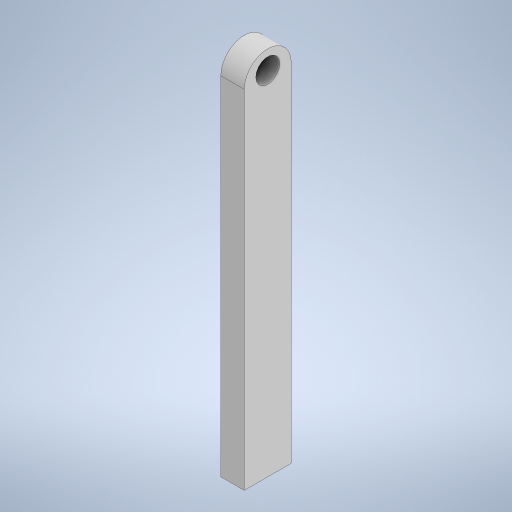
# Autodesk Inventor part: HolzHalter
Saved by Autodesk Inventor 2023 (Build 270158000, 158)
## iProperties
Created: 2024-02-23
Part Number: HolzHalter
Material: Generisch
Document SubType Name: Modeling
Designer: phili
Density: 1 g/cm^3
Appearance: Vorgabe
Author: phili
Autodesk Inventor part; units mm, degrees
ref_plane "YZ Plane" through (0, 0, 0) normal (1, 0, 0) x (0, 1, 0)
ref_plane "XZ Plane" through (0, 0, 0) normal (0, 1, 0) x (-1, 0, 0)
ref_plane "XY Plane" through (0, 0, 0) normal (0, 0, 1) x (1, 0, 0)
sketch "Skizze1" plane through (0, 0, 0) normal (1, 0, 0) x (0, 1, 0)
  line L0 (0, 0) -> (158, 0)
  line L1 (158, 0) -> (158, -20)
  line L2 (158, -20) -> (0, -20)
  line L3 (0, -20) -> (0, 0)
  dimension "d0" = 158
  dimension "d1" = 20
  constraints: 8 end point, 2 parallel, 1 horizontal, 1 perpendicular
  measures "d0" distance of L1.end L2.end
  measures "d1" distance of L0.end L1.end
extrude "Extrusion1" add sketch "Skizze1" along normal blind 10
sketch "Skizze2" plane through (10, 0, 0) normal (1, 0, 0) x (0, 0, -1)
  line L0 (0, 0) -> (20, 0) projected
  line L1 (20, 0) -> (20, 158) projected
  point P0 (10, 150)
  dimension "d11" = 150
  dimension "d12" = 10
  measures "d11" distance from line of point (10, 150) L0
  measures "d12" distance from line of L1 point (10, 150)
hole "Bohrung1" at (10, 150, -10) direction (-1, 0, 0) diameter 10.2 end through all
fillet "Rundung1" radius 10 2 edges at (5, 158, 0) (5, 158, -20)
